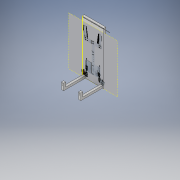
# Autodesk Inventor part: Pretend this is a harness
Saved by Autodesk Inventor 2018 (Build 220112000, 112)
## iProperties
Created: 2018-12-30
Part Number: Pretend this is a harness
Material: Generic
Document SubType Name: Modeling
Designer: maste
Density: 1 g/cm^3
Appearance: Default
Author: maste
Autodesk Inventor part; units mm, degrees
(part 1 of 4)
ref_plane "YZ Plane" through (0, 0, 0) normal (1, 0, 0) x (0, 1, 0)
ref_plane "XZ Plane" through (0, 0, 0) normal (0, 1, 0) x (-1, 0, 0)
ref_plane "XY Plane" through (0, 0, 0) normal (0, 0, 1) x (1, 0, 0)
sketch "Sketch1" plane through (0, 0, 0) normal (0, 0, 1) x (1, 0, 0)
  line L0 (0, 0) -> (250.7996, 0)
  line L1 (250.7996, 0) -> (250.7996, 609.6)
  line L2 (250.7996, 609.6) -> (0, 609.6)
  line L3 (0, 609.6) -> (0, 0)
  dimension "d0" = 250.7996
  dimension "d1" = 609.6
  constraints: 8 end point, 2 parallel, 1 horizontal, 1 perpendicular
  measures "d0" distance of L2.end L1.end
  measures "d1" distance of L1.end L0.end
extrude "Extrusion1" add sketch "Sketch1" along normal blind 25.4
sketch "Sketch2" plane through (0, 0, 25.4) normal (0, 0, 1) x (1, 0, 0)
  line L0 (0, 0) -> (25.4, 0) construction
  line L1 (0, 0) -> (250.7996, 0) construction
  line L2 (250.7996, 0) -> (225.3996, 0) construction
  line L3 (25.4, 0) -> (38.1, 0) construction
  line L4 (38.1, 0) -> (38.1, 25.4)
  line L5 (38.1, 25.4) -> (12.7, 25.4)
  line L6 (12.7, 25.4) -> (12.7, 0)
  line L7 (38.1, 0) -> (12.7, 0)
  line L8 (125.3998, 0) -> (125.3998, 65.8359) construction
  line L9 (250.7996, 0) -> (225.3996, 0) construction
  line L10 (250.7996, 0) -> (0, 0) construction
  line L11 (225.3996, 0) -> (212.6996, 0) construction
  line L12 (212.6996, 0) -> (212.6996, 25.4)
  line L13 (212.6996, 25.4) -> (238.0996, 25.4)
  line L14 (238.0996, 25.4) -> (238.0996, 0)
  line L15 (212.6996, 0) -> (238.0996, 0)
  dimension "d4" = 25.4
  dimension "d5" = 25.4
  dimension "d6" = 12.7
  dimension "d7" = 25.4
  dimension "d8" = 25.4
  constraints: 30 end point, 7 point on line, 6 symmetric about line, 3 perpendicular, 1 collinear, 1 midpoint, 1 vertical
  measures "d4" distance of L0.start L0.end
  measures "d5" distance of L1.end L2.end
  measures "d6" distance of L0.end L3.end
  measures "d7" distance of L3.end L4.end
  measures "d8" distance of L4.end L5.end
extrude "Extrusion2" add sketch "Sketch2" along normal blind 254
sketch "Sketch3" plane through (212.6996, 25.4, 25.4) normal (0, 1, 0) x (1, 0, 0)
  line L0 (-199.9996, -254) -> (-174.5996, -254) projected
  line L1 (-199.9996, -254) -> (-174.5996, -254)
  line L2 (-174.5996, -254) -> (-174.5996, -228.6)
  line L3 (-174.5996, -228.6) -> (-199.9996, -228.6)
  line L4 (-199.9996, -228.6) -> (-199.9996, -254)
  line L5 (0, -254) -> (25.4, -254) projected
  line L6 (25.4, 0) -> (25.4, -254) projected
  line L7 (0, -254) -> (25.4, -254)
  line L8 (25.4, -254) -> (25.4, -228.6)
  line L9 (25.4, -228.6) -> (0, -228.6)
  line L10 (0, -228.6) -> (0, -254)
  point P0 (-212.6996, 25.4)
  dimension "d11" = 25.4
  dimension "d12" = 25.4
  constraints: 16 end point, 4 parallel, 2 horizontal, 2 perpendicular, 2 point on line
  measures "d11" distance of L3.end L2.end
  measures "d12" distance of L2.end L1.end
extrude "Extrusion3" add sketch "Sketch3" along normal blind 50.8
sketch "Sketch4" plane through (0, 0, 279.4) normal (0, 0, 1) x (1, 0, 0)
  line L0 (38.1, 76.2) -> (12.7, 76.2) construction
  line L1 (25.4, 76.2) -> (25.4, 63.5) construction
  line L2 (25.4, 63.5) -> (25.4, 50.8) construction
  line L3 (38.1, 0) -> (212.6996, 0) construction
  line L4 (125.3998, 0) -> (125.3998, 112.4293) construction
  circle A0 centre (25.4, 50.8) radius 2.5797
  circle A1 centre (25.4, 63.5) radius 2.5797
  line L5 (212.6996, 76.2) -> (238.0996, 76.2) construction
  line L6 (225.3996, 76.2) -> (225.3996, 63.5) construction
  line L7 (225.3996, 63.5) -> (225.3996, 50.8) construction
  circle A2 centre (225.3996, 50.8) radius 2.5797
  circle A3 centre (225.3996, 63.5) radius 2.5797
  point P0 (0, 0)
  dimension "d15" = 12.7
  dimension "d16" = 12.7
  dimension "d17" = 5.1594
  constraints: 12 end point, 7 symmetric about line, 4 centre point, 4 coincident, 2 midpoint, 2 point on line, 2 vertical, 2 other
  measures "d15" distance of L1.start L1.end
  measures "d16" distance of L1.end L2.end
  measures "d17" diameter of A0
extrude "Extrusion4" cut sketch "Sketch4" against normal blind 50.8
sketch "Sketch5" plane through (0, 0, 25.4) normal (0, 0, 1) x (1, 0, 0)
  line L0 (0, 609.6) -> (0, 0) projected
  line L1 (-154.3078, 564.0513) -> (411.5707, 564.0513) construction
  line L2 (411.5707, 564.0513) -> (411.5707, -1.8272) construction
  line L3 (411.5707, -1.8272) -> (-154.3078, -1.8272) construction
  line L4 (-154.3078, -1.8272) -> (-154.3078, 564.0513) construction
  constraints: 2 end point, 2 other
sketch "Sketch6" plane through (0, 0, 25.4) normal (0, 0, 1) x (1, 0, 0)
  line L0 (9.9083, 603.5632) -> (254.2523, 603.5632) construction
  line L1 (254.2523, 603.5632) -> (254.2523, 561.4608) construction
  line L2 (254.2523, 561.4608) -> (9.9083, 561.4608) construction
  line L3 (9.9083, 561.4608) -> (9.9083, 603.5632) construction
  line L4 (11.9831, 600.3596) -> (11.5977, 600.3596)
  line L5 (11.5977, 600.3596) -> (11.5977, 601.6637)
  spline S0 degree 2 poles (11.5977, 601.6637) (11.5977, 601.8218) (11.5681, 602.0935) (11.5236, 602.175) knots 0 0 0 1 2 2 2
  spline S1 degree 2 poles (11.5236, 602.175) (11.4767, 602.2615) (11.3088, 602.3455) (11.1655, 602.3455) knots 0 0 0 1 2 2 2
  spline S2 degree 2 poles (11.1655, 602.3455) (11.0222, 602.3455) (10.7184, 602.1923) (10.5727, 602.0688) knots 0 0 0 1 2 2 2
  line L6 (10.5727, 602.0688) -> (10.5727, 600.3596)
  line L7 (10.5727, 600.3596) -> (10.1874, 600.3596)
  line L8 (10.1874, 600.3596) -> (10.1874, 603.5434)
  line L9 (10.1874, 603.5434) -> (10.5727, 603.5434)
  line L10 (10.5727, 603.5434) -> (10.5727, 602.3924)
  spline S3 degree 2 poles (10.5727, 602.3924) (10.7456, 602.548) (11.079, 602.711) (11.2668, 602.711) knots 0 0 0 1 2 2 2
  spline S4 degree 2 poles (11.2668, 602.711) (11.6027, 602.711) (11.9831, 602.2664) (11.9831, 601.844) knots 0 0 0 1 2 2 2
  line L11 (11.9831, 601.844) -> (11.9831, 600.3596)
  spline S5 degree 2 poles (13.2156, 600.3151) (12.9019, 600.3151) (12.5487, 600.6733) (12.5487, 601.061) knots 0 0 0 1 2 2 2
  line L12 (12.5487, 601.061) -> (12.5487, 602.3282)
  line L13 (12.5487, 602.3282) -> (12.2893, 602.3282)
  line L14 (12.2893, 602.3282) -> (12.2893, 602.6468)
  line L15 (12.2893, 602.6468) -> (12.5487, 602.6468)
  line L16 (12.5487, 602.6468) -> (12.5487, 603.3038)
  line L17 (12.5487, 603.3038) -> (12.934, 603.3038)
  line L18 (12.934, 603.3038) -> (12.934, 602.6468)
  line L19 (12.934, 602.6468) -> (13.6429, 602.6468)
  line L20 (13.6429, 602.6468) -> (13.6429, 602.3282)
  line L21 (13.6429, 602.3282) -> (12.934, 602.3282)
  line L22 (12.934, 602.3282) -> (12.934, 601.2389)
  spline S6 degree 2 poles (12.934, 601.2389) (12.934, 601.066) (12.9464, 600.8758) (12.9884, 600.7943) knots 0 0 0 1 2 2 2
  spline S7 degree 2 poles (12.9884, 600.7943) (13.0229, 600.7227) (13.1786, 600.651) (13.3119, 600.651) knots 0 0 0 1 2 2 2
  spline S8 degree 2 poles (13.3119, 600.651) (13.4058, 600.651) (13.5812, 600.7078) (13.6207, 600.7251) knots 0 0 0 1 2 2 2
  line L23 (13.6207, 600.7251) -> (13.6429, 600.7251)
  line L24 (13.6429, 600.7251) -> (13.6429, 600.3793)
  spline S9 degree 2 poles (13.6429, 600.3793) (13.5342, 600.3497) (13.3119, 600.3151) (13.2156, 600.3151) knots 0 0 0 1 2 2 2
  spline S10 degree 2 poles (14.6186, 600.3151) (14.3049, 600.3151) (13.9517, 600.6733) (13.9517, 601.061) knots 0 0 0 1 2 2 2
  line L25 (13.9517, 601.061) -> (13.9517, 602.3282)
  line L26 (13.9517, 602.3282) -> (13.6923, 602.3282)
  line L27 (13.6923, 602.3282) -> (13.6923, 602.6468)
  line L28 (13.6923, 602.6468) -> (13.9517, 602.6468)
  line L29 (13.9517, 602.6468) -> (13.9517, 603.3038)
  line L30 (13.9517, 603.3038) -> (14.337, 603.3038)
  line L31 (14.337, 603.3038) -> (14.337, 602.6468)
  line L32 (14.337, 602.6468) -> (15.0459, 602.6468)
  line L33 (15.0459, 602.6468) -> (15.0459, 602.3282)
  line L34 (15.0459, 602.3282) -> (14.337, 602.3282)
  line L35 (14.337, 602.3282) -> (14.337, 601.2389)
  spline S11 degree 2 poles (14.337, 601.2389) (14.337, 601.066) (14.3493, 600.8758) (14.3913, 600.7943) knots 0 0 0 1 2 2 2
  spline S12 degree 2 poles (14.3913, 600.7943) (14.4259, 600.7227) (14.5815, 600.651) (14.7149, 600.651) knots 0 0 0 1 2 2 2
  spline S13 degree 2 poles (14.7149, 600.651) (14.8088, 600.651) (14.9841, 600.7078) (15.0237, 600.7251) knots 0 0 0 1 2 2 2
  line L36 (15.0237, 600.7251) -> (15.0459, 600.7251)
  line L37 (15.0459, 600.7251) -> (15.0459, 600.3793)
  spline S14 degree 2 poles (15.0459, 600.3793) (14.9372, 600.3497) (14.7149, 600.3151) (14.6186, 600.3151) knots 0 0 0 1 2 2 2
  spline S15 degree 2 poles (17.2467, 601.5649) (17.2467, 600.9919) (16.7008, 600.3151) (16.2834, 600.3151) knots 0 0 0 1 2 2 2
  spline S16 degree 2 poles (16.2834, 600.3151) (16.1129, 600.3151) (15.8511, 600.3941) (15.7153, 600.4757) knots 0 0 0 1 2 2 2
  line L38 (15.7153, 600.4757) -> (15.7153, 599.5173)
  line L39 (15.7153, 599.5173) -> (15.3299, 599.5173)
  line L40 (15.3299, 599.5173) -> (15.3299, 602.6468)
  line L41 (15.3299, 602.6468) -> (15.7153, 602.6468)
  line L42 (15.7153, 602.6468) -> (15.7153, 602.4072)
  spline S17 degree 2 poles (15.7153, 602.4072) (15.8585, 602.5381) (16.2093, 602.711) (16.4143, 602.711) knots 0 0 0 1 2 2 2
  spline S18 degree 2 poles (16.4143, 602.711) (16.807, 602.711) (17.2467, 602.0886) (17.2467, 601.5649) knots 0 0 0 1 2 2 2
  spline S19 degree 2 poles (16.849, 601.5205) (16.849, 601.9132) (16.5995, 602.3455) (16.3204, 602.3455) knots 0 0 0 1 2 2 2
  spline S20 degree 2 poles (16.3204, 602.3455) (16.1574, 602.3455) (15.8511, 602.1997) (15.7153, 602.0861) knots 0 0 0 1 2 2 2
  line L43 (15.7153, 602.0861) -> (15.7153, 600.7869)
  spline S21 degree 2 poles (15.7153, 600.7869) (15.8659, 600.7152) (16.0808, 600.6609) (16.2191, 600.6609) knots 0 0 0 1 2 2 2
  spline S22 degree 2 poles (16.2191, 600.6609) (16.518, 600.6609) (16.849, 601.1006) (16.849, 601.5205) knots 0 0 0 1 2 2 2
  spline S23 degree 2 poles (18.2643, 600.3052) (18.0346, 600.3052) (17.6369, 600.4287) (17.506, 600.4979) knots 0 0 0 1 2 2 2
  line L44 (17.506, 600.4979) -> (17.506, 600.9301)
  line L45 (17.506, 600.9301) -> (17.5258, 600.9301)
  spline S24 degree 2 poles (17.5258, 600.9301) (17.5752, 600.8906) (17.7086, 600.7968) (17.8197, 600.7449) knots 0 0 0 1 2 2 2
  spline S25 degree 2 poles (17.8197, 600.7449) (17.916, 600.698) (18.1532, 600.6288) (18.2791, 600.6288) knots 0 0 0 1 2 2 2
  spline S26 degree 2 poles (18.2791, 600.6288) (18.3705, 600.6288) (18.5805, 600.6708) (18.6299, 600.7054) knots 0 0 0 1 2 2 2
  spline S27 degree 2 poles (18.6299, 600.7054) (18.7015, 600.7523) (18.7657, 600.8585) (18.7657, 600.9672) knots 0 0 0 1 2 2 2
  spline S28 degree 2 poles (18.7657, 600.9672) (18.7657, 601.103) (18.6175, 601.2438) (18.4273, 601.2908) knots 0 0 0 1 2 2 2
  spline S29 degree 2 poles (18.4273, 601.2908) (18.3532, 601.3081) (18.1161, 601.3575) (18.0148, 601.3846) knots 0 0 0 1 2 2 2
  spline S30 degree 2 poles (18.0148, 601.3846) (17.753, 601.4612) (17.5159, 601.7774) (17.5159, 602.0021) knots 0 0 0 1 2 2 2
  spline S31 degree 2 poles (17.5159, 602.0021) (17.5159, 602.3133) (17.9827, 602.7011) (18.3681, 602.7011) knots 0 0 0 1 2 2 2
  spline S32 degree 2 poles (18.3681, 602.7011) (18.5582, 602.7011) (18.9436, 602.6073) (19.0745, 602.5356) knots 0 0 0 1 2 2 2
  line L46 (19.0745, 602.5356) -> (19.0745, 602.1232)
  line L47 (19.0745, 602.1232) -> (19.0547, 602.1232)
  spline S33 degree 2 poles (19.0547, 602.1232) (18.9065, 602.2417) (18.5459, 602.3776) (18.3606, 602.3776) knots 0 0 0 1 2 2 2
  spline S34 degree 2 poles (18.3606, 602.3776) (18.1705, 602.3776) (17.9086, 602.217) (17.9086, 602.0565) knots 0 0 0 1 2 2 2
  spline S35 degree 2 poles (17.9086, 602.0565) (17.9086, 601.9107) (18.0642, 601.7699) (18.2371, 601.7255) knots 0 0 0 1 2 2 2
  spline S36 degree 2 poles (18.2371, 601.7255) (18.3211, 601.7033) (18.5335, 601.6588) (18.6496, 601.6316) knots 0 0 0 1 2 2 2
  spline S37 degree 2 poles (18.6496, 601.6316) (18.9016, 601.5674) (19.1585, 601.2735) (19.1585, 601.0191) knots 0 0 0 1 2 2 2
  spline S38 degree 2 poles (19.1585, 601.0191) (19.1585, 600.8709) (19.0424, 600.609) (18.9288, 600.5127) knots 0 0 0 1 2 2 2
  spline S39 degree 2 poles (18.9288, 600.5127) (18.8077, 600.4114) (18.499, 600.3052) (18.2643, 600.3052) knots 0 0 0 1 2 2 2
  line L48 (20.223, 600.3596) -> (19.734, 600.3596)
  line L49 (19.734, 600.3596) -> (19.734, 600.9425)
  line L50 (19.734, 600.9425) -> (20.223, 600.9425)
  line L51 (20.223, 600.9425) -> (20.223, 600.3596)
  line L52 (20.223, 602.0639) -> (19.734, 602.0639)
  line L53 (19.734, 602.0639) -> (19.734, 602.6468)
  line L54 (19.734, 602.6468) -> (20.223, 602.6468)
  line L55 (20.223, 602.6468) -> (20.223, 602.0639)
  line L56 (22.2089, 603.5434) -> (21.0159, 599.6976)
  line L57 (21.0159, 599.6976) -> (20.6701, 599.6976)
  line L58 (20.6701, 599.6976) -> (21.8582, 603.5434)
  line L59 (21.8582, 603.5434) -> (22.2089, 603.5434)
  line L60 (23.812, 603.5434) -> (22.619, 599.6976)
  line L61 (22.619, 599.6976) -> (22.2732, 599.6976)
  line L62 (22.2732, 599.6976) -> (23.4612, 603.5434)
  line L63 (23.4612, 603.5434) -> (23.812, 603.5434)
  line L64 (26.9761, 602.6468) -> (26.3956, 600.3596)
  line L65 (26.3956, 600.3596) -> (26.0399, 600.3596)
  line L66 (26.0399, 600.3596) -> (25.4817, 602.1232)
  line L67 (25.4817, 602.1232) -> (24.926, 600.3596)
  line L68 (24.926, 600.3596) -> (24.5727, 600.3596)
  line L69 (24.5727, 600.3596) -> (23.9873, 602.6468)
  line L70 (23.9873, 602.6468) -> (24.3875, 602.6468)
  line L71 (24.3875, 602.6468) -> (24.7926, 600.8758)
  line L72 (24.7926, 600.8758) -> (25.3335, 602.6468)
  line L73 (25.3335, 602.6468) -> (25.6521, 602.6468)
  line L74 (25.6521, 602.6468) -> (26.2079, 600.8758)
  line L75 (26.2079, 600.8758) -> (26.5883, 602.6468)
  line L76 (26.5883, 602.6468) -> (26.9761, 602.6468)
  line L77 (30.0858, 602.6468) -> (29.5054, 600.3596)
  line L78 (29.5054, 600.3596) -> (29.1497, 600.3596)
  line L79 (29.1497, 600.3596) -> (28.5915, 602.1232)
  line L80 (28.5915, 602.1232) -> (28.0357, 600.3596)
  line L81 (28.0357, 600.3596) -> (27.6825, 600.3596)
  line L82 (27.6825, 600.3596) -> (27.0971, 602.6468)
  line L83 (27.0971, 602.6468) -> (27.4972, 602.6468)
  line L84 (27.4972, 602.6468) -> (27.9023, 600.8758)
  line L85 (27.9023, 600.8758) -> (28.4433, 602.6468)
  line L86 (28.4433, 602.6468) -> (28.7619, 602.6468)
  line L87 (28.7619, 602.6468) -> (29.3176, 600.8758)
  line L88 (29.3176, 600.8758) -> (29.698, 602.6468)
  line L89 (29.698, 602.6468) -> (30.0858, 602.6468)
  line L90 (33.1956, 602.6468) -> (32.6151, 600.3596)
  line L91 (32.6151, 600.3596) -> (32.2594, 600.3596)
  line L92 (32.2594, 600.3596) -> (31.7012, 602.1232)
  line L93 (31.7012, 602.1232) -> (31.1455, 600.3596)
  line L94 (31.1455, 600.3596) -> (30.7922, 600.3596)
  line L95 (30.7922, 600.3596) -> (30.2068, 602.6468)
  line L96 (30.2068, 602.6468) -> (30.607, 602.6468)
  line L97 (30.607, 602.6468) -> (31.0121, 600.8758)
  line L98 (31.0121, 600.8758) -> (31.553, 602.6468)
  line L99 (31.553, 602.6468) -> (31.8716, 602.6468)
  line L100 (31.8716, 602.6468) -> (32.4274, 600.8758)
  line L101 (32.4274, 600.8758) -> (32.8078, 602.6468)
  line L102 (32.8078, 602.6468) -> (33.1956, 602.6468)
  line L103 (34.1317, 600.3596) -> (33.6426, 600.3596)
  line L104 (33.6426, 600.3596) -> (33.6426, 600.9425)
  line L105 (33.6426, 600.9425) -> (34.1317, 600.9425)
  line L106 (34.1317, 600.9425) -> (34.1317, 600.3596)
  spline S40 degree 2 poles (36.0781, 600.6016) (36.0311, 600.567) (35.8731, 600.4435) (35.799, 600.4065) knots 0 0 0 1 2 2 2
  spline S41 degree 2 poles (35.799, 600.4065) (35.6977, 600.3522) (35.5075, 600.2953) (35.3346, 600.2953) knots 0 0 0 1 2 2 2
  spline S42 degree 2 poles (35.3346, 600.2953) (35.1938, 600.2953) (34.9394, 600.4016) (34.8431, 600.4979) knots 0 0 0 1 2 2 2
  spline S43 degree 2 poles (34.8431, 600.4979) (34.7517, 600.5917) (34.6405, 600.8684) (34.6405, 601.0215) knots 0 0 0 1 2 2 2
  spline S44 degree 2 poles (34.6405, 601.0215) (34.6405, 601.2587) (34.8406, 601.5946) (35.058, 601.6909) knots 0 0 0 1 2 2 2
  spline S45 degree 2 poles (35.058, 601.6909) (35.2506, 601.7798) (35.7743, 601.8465) (36.0781, 601.8638) knots 0 0 0 1 2 2 2
  line L107 (36.0781, 601.8638) -> (36.0781, 601.9379)
  spline S46 degree 2 poles (36.0781, 601.9379) (36.0781, 602.0713) (35.9966, 602.2368) (35.9225, 602.2837) knots 0 0 0 1 2 2 2
  spline S47 degree 2 poles (35.9225, 602.2837) (35.8484, 602.3306) (35.6359, 602.3603) (35.5223, 602.3603) knots 0 0 0 1 2 2 2
  spline S48 degree 2 poles (35.5223, 602.3603) (35.3889, 602.3603) (35.0283, 602.2812) (34.848, 602.2047) knots 0 0 0 1 2 2 2
  line L108 (34.848, 602.2047) -> (34.8258, 602.2047)
  line L109 (34.8258, 602.2047) -> (34.8258, 602.5974)
  spline S49 degree 2 poles (34.8258, 602.5974) (34.932, 602.627) (35.3297, 602.7011) (35.5248, 602.7011) knots 0 0 0 1 2 2 2
  spline S50 degree 2 poles (35.5248, 602.7011) (35.7619, 602.7011) (36.0855, 602.627) (36.2139, 602.5307) knots 0 0 0 1 2 2 2
  spline S51 degree 2 poles (36.2139, 602.5307) (36.3399, 602.4368) (36.4634, 602.138) (36.4634, 601.9231) knots 0 0 0 1 2 2 2
  line L110 (36.4634, 601.9231) -> (36.4634, 600.3596)
  line L111 (36.4634, 600.3596) -> (36.0781, 600.3596)
  line L112 (36.0781, 600.3596) -> (36.0781, 600.6016)
  line L113 (36.0781, 600.9227) -> (36.0781, 601.5575)
  spline S52 degree 2 poles (36.0781, 601.5575) (35.9398, 601.5452) (35.5223, 601.5032) (35.3914, 601.4637) knots 0 0 0 1 2 2 2
  spline S53 degree 2 poles (35.3914, 601.4637) (35.2383, 601.4167) (35.0382, 601.2216) (35.0382, 601.0487) knots 0 0 0 1 2 2 2
  spline S54 degree 2 poles (35.0382, 601.0487) (35.0382, 600.8511) (35.2605, 600.651) (35.4729, 600.651) knots 0 0 0 1 2 2 2
  spline S55 degree 2 poles (35.4729, 600.651) (35.6532, 600.651) (35.9496, 600.8066) (36.0781, 600.9227) knots 0 0 0 1 2 2 2
  line L114 (39.5978, 600.3596) -> (39.5978, 601.6835)
  spline S56 degree 2 poles (39.5978, 601.6835) (39.5978, 601.8416) (39.5731, 602.1108) (39.5336, 602.1849) knots 0 0 0 1 2 2 2
  spline S57 degree 2 poles (39.5336, 602.1849) (39.4941, 602.2664) (39.3434, 602.3455) (39.2125, 602.3455) knots 0 0 0 1 2 2 2
  spline S58 degree 2 poles (39.2125, 602.3455) (39.094, 602.3455) (38.8223, 602.1997) (38.679, 602.0614) knots 0 0 0 1 2 2 2
  spline S59 degree 2 poles (38.679, 602.0614) (38.6815, 602.0268) (38.6864, 601.9305) (38.6864, 601.8663) knots 0 0 0 1 2 2 2
  line L115 (38.6864, 601.8663) -> (38.6864, 600.3596)
  line L116 (38.6864, 600.3596) -> (38.3011, 600.3596)
  line L117 (38.3011, 600.3596) -> (38.3011, 601.6835)
  spline S60 degree 2 poles (38.3011, 601.6835) (38.3011, 601.8416) (38.2764, 602.1108) (38.2369, 602.1849) knots 0 0 0 1 2 2 2
  spline S61 degree 2 poles (38.2369, 602.1849) (38.1973, 602.2664) (38.0467, 602.3455) (37.9158, 602.3455) knots 0 0 0 1 2 2 2
  spline S62 degree 2 poles (37.9158, 602.3455) (37.7923, 602.3455) (37.5181, 602.1898) (37.3897, 602.0688) knots 0 0 0 1 2 2 2
  line L118 (37.3897, 602.0688) -> (37.3897, 600.3596)
  line L119 (37.3897, 600.3596) -> (37.0043, 600.3596)
  line L120 (37.0043, 600.3596) -> (37.0043, 602.6468)
  line L121 (37.0043, 602.6468) -> (37.3897, 602.6468)
  line L122 (37.3897, 602.6468) -> (37.3897, 602.3949)
  spline S63 degree 2 poles (37.3897, 602.3949) (37.5403, 602.5455) (37.8367, 602.711) (38.0146, 602.711) knots 0 0 0 1 2 2 2
  spline S64 degree 2 poles (38.0146, 602.711) (38.2171, 602.711) (38.5308, 602.5258) (38.6123, 602.3158) knots 0 0 0 1 2 2 2
  spline S65 degree 2 poles (38.6123, 602.3158) (38.7877, 602.5109) (39.1187, 602.711) (39.3113, 602.711) knots 0 0 0 1 2 2 2
  spline S66 degree 2 poles (39.3113, 602.711) (39.4595, 602.711) (39.7016, 602.6196) (39.7905, 602.5159) knots 0 0 0 1 2 2 2
  spline S67 degree 2 poles (39.7905, 602.5159) (39.8819, 602.4121) (39.9832, 602.1009) (39.9832, 601.8663) knots 0 0 0 1 2 2 2
  line L123 (39.9832, 601.8663) -> (39.9832, 600.3596)
  line L124 (39.9832, 600.3596) -> (39.5978, 600.3596)
  spline S68 degree 2 poles (41.7986, 600.6016) (41.7517, 600.567) (41.5936, 600.4435) (41.5195, 600.4065) knots 0 0 0 1 2 2 2
  spline S69 degree 2 poles (41.5195, 600.4065) (41.4182, 600.3522) (41.2281, 600.2953) (41.0552, 600.2953) knots 0 0 0 1 2 2 2
  spline S70 degree 2 poles (41.0552, 600.2953) (40.9144, 600.2953) (40.66, 600.4016) (40.5636, 600.4979) knots 0 0 0 1 2 2 2
  spline S71 degree 2 poles (40.5636, 600.4979) (40.4722, 600.5917) (40.3611, 600.8684) (40.3611, 601.0215) knots 0 0 0 1 2 2 2
  spline S72 degree 2 poles (40.3611, 601.0215) (40.3611, 601.2587) (40.5612, 601.5946) (40.7785, 601.6909) knots 0 0 0 1 2 2 2
  spline S73 degree 2 poles (40.7785, 601.6909) (40.9712, 601.7798) (41.4948, 601.8465) (41.7986, 601.8638) knots 0 0 0 1 2 2 2
  line L125 (41.7986, 601.8638) -> (41.7986, 601.9379)
  spline S74 degree 2 poles (41.7986, 601.9379) (41.7986, 602.0713) (41.7171, 602.2368) (41.643, 602.2837) knots 0 0 0 1 2 2 2
  spline S75 degree 2 poles (41.643, 602.2837) (41.5689, 602.3306) (41.3565, 602.3603) (41.2429, 602.3603) knots 0 0 0 1 2 2 2
  spline S76 degree 2 poles (41.2429, 602.3603) (41.1095, 602.3603) (40.7489, 602.2812) (40.5686, 602.2047) knots 0 0 0 1 2 2 2
  line L126 (40.5686, 602.2047) -> (40.5463, 602.2047)
  line L127 (40.5463, 602.2047) -> (40.5463, 602.5974)
  spline S77 degree 2 poles (40.5463, 602.5974) (40.6525, 602.627) (41.0502, 602.7011) (41.2453, 602.7011) knots 0 0 0 1 2 2 2
  spline S78 degree 2 poles (41.2453, 602.7011) (41.4825, 602.7011) (41.806, 602.627) (41.9345, 602.5307) knots 0 0 0 1 2 2 2
  spline S79 degree 2 poles (41.9345, 602.5307) (42.0605, 602.4368) (42.184, 602.138) (42.184, 601.9231) knots 0 0 0 1 2 2 2
  line L128 (42.184, 601.9231) -> (42.184, 600.3596)
  line L129 (42.184, 600.3596) -> (41.7986, 600.3596)
  line L130 (41.7986, 600.3596) -> (41.7986, 600.6016)
  line L131 (41.7986, 600.9227) -> (41.7986, 601.5575)
  spline S80 degree 2 poles (41.7986, 601.5575) (41.6603, 601.5452) (41.2429, 601.5032) (41.112, 601.4637) knots 0 0 0 1 2 2 2
  spline S81 degree 2 poles (41.112, 601.4637) (40.9588, 601.4167) (40.7588, 601.2216) (40.7588, 601.0487) knots 0 0 0 1 2 2 2
  spline S82 degree 2 poles (40.7588, 601.0487) (40.7588, 600.8511) (40.9811, 600.651) (41.1935, 600.651) knots 0 0 0 1 2 2 2
  spline S83 degree 2 poles (41.1935, 600.651) (41.3738, 600.651) (41.6702, 600.8066) (41.7986, 600.9227) knots 0 0 0 1 2 2 2
  line L132 (44.2267, 600.3596) -> (42.547, 600.3596)
  line L133 (42.547, 600.3596) -> (42.547, 600.6461)
  line L134 (42.547, 600.6461) -> (43.7425, 602.3306)
  line L135 (43.7425, 602.3306) -> (42.5964, 602.3306)
  line L136 (42.5964, 602.3306) -> (42.5964, 602.6468)
  line L137 (42.5964, 602.6468) -> (44.2044, 602.6468)
  line L138 (44.2044, 602.6468) -> (44.2044, 602.3726)
  line L139 (44.2044, 602.3726) -> (43.004, 600.6831)
  line L140 (43.004, 600.6831) -> (44.2267, 600.6831)
  line L141 (44.2267, 600.6831) -> (44.2267, 600.3596)
  spline S84 degree 2 poles (46.467, 601.5032) (46.467, 600.9252) (45.9112, 600.2953) (45.4468, 600.2953) knots 0 0 0 1 2 2 2
  spline S85 degree 2 poles (45.4468, 600.2953) (44.9701, 600.2953) (44.4243, 600.945) (44.4243, 601.5032) knots 0 0 0 1 2 2 2
  spline S86 degree 2 poles (44.4243, 601.5032) (44.4243, 602.0762) (44.9874, 602.711) (45.4468, 602.711) knots 0 0 0 1 2 2 2
  spline S87 degree 2 poles (45.4468, 602.711) (45.9112, 602.711) (46.467, 602.0787) (46.467, 601.5032) knots 0 0 0 1 2 2 2
  spline S88 degree 2 poles (46.0693, 601.5032) (46.0693, 601.9478) (45.7457, 602.38) (45.4468, 602.38) knots 0 0 0 1 2 2 2
  spline S89 degree 2 poles (45.4468, 602.38) (45.148, 602.38) (44.8219, 601.9478) (44.8219, 601.5032) knots 0 0 0 1 2 2 2
  spline S90 degree 2 poles (44.8219, 601.5032) (44.8219, 601.0709) (45.148, 600.6263) (45.4468, 600.6263) knots 0 0 0 1 2 2 2
  spline S91 degree 2 poles (45.4468, 600.6263) (45.7432, 600.6263) (46.0693, 601.0635) (46.0693, 601.5032) knots 0 0 0 1 2 2 2
  line L142 (48.6579, 600.3596) -> (48.2725, 600.3596)
  line L143 (48.2725, 600.3596) -> (48.2725, 601.6637)
  spline S92 degree 2 poles (48.2725, 601.6637) (48.2725, 601.8218) (48.2429, 602.0935) (48.1984, 602.175) knots 0 0 0 1 2 2 2
  spline S93 degree 2 poles (48.1984, 602.175) (48.1515, 602.2615) (47.9836, 602.3455) (47.8403, 602.3455) knots 0 0 0 1 2 2 2
  spline S94 degree 2 poles (47.8403, 602.3455) (47.697, 602.3455) (47.3932, 602.1923) (47.2475, 602.0688) knots 0 0 0 1 2 2 2
  line L144 (47.2475, 602.0688) -> (47.2475, 600.3596)
  line L145 (47.2475, 600.3596) -> (46.8622, 600.3596)
  line L146 (46.8622, 600.3596) -> (46.8622, 602.6468)
  line L147 (46.8622, 602.6468) -> (47.2475, 602.6468)
  line L148 (47.2475, 602.6468) -> (47.2475, 602.3924)
  spline S95 degree 2 poles (47.2475, 602.3924) (47.4204, 602.548) (47.7538, 602.711) (47.9416, 602.711) knots 0 0 0 1 2 2 2
  spline S96 degree 2 poles (47.9416, 602.711) (48.2775, 602.711) (48.6579, 602.2664) (48.6579, 601.844) knots 0 0 0 1 2 2 2
  line L149 (48.6579, 601.844) -> (48.6579, 600.3596)
  line L150 (49.7965, 600.3596) -> (49.3075, 600.3596)
  line L151 (49.3075, 600.3596) -> (49.3075, 600.9425)
  line L152 (49.3075, 600.9425) -> (49.7965, 600.9425)
  line L153 (49.7965, 600.9425) -> (49.7965, 600.3596)
  spline S97 degree 2 poles (51.3774, 600.3077) (51.1402, 600.3077) (50.7475, 600.4534) (50.6067, 600.6016) knots 0 0 0 1 2 2 2
  spline S98 degree 2 poles (50.6067, 600.6016) (50.4659, 600.7474) (50.3103, 601.1969) (50.3103, 601.4982) knots 0 0 0 1 2 2 2
  spline S99 degree 2 poles (50.3103, 601.4982) (50.3103, 601.7996) (50.4709, 602.2392) (50.6067, 602.3874) knots 0 0 0 1 2 2 2
  spline S100 degree 2 poles (50.6067, 602.3874) (50.7426, 602.5381) (51.1452, 602.6987) (51.3774, 602.6987) knots 0 0 0 1 2 2 2
  spline S101 degree 2 poles (51.3774, 602.6987) (51.5651, 602.6987) (51.9158, 602.5925) (52.0517, 602.5233) knots 0 0 0 1 2 2 2
  line L154 (52.0517, 602.5233) -> (52.0517, 602.091)
  line L155 (52.0517, 602.091) -> (52.0294, 602.091)
  spline S102 degree 2 poles (52.0294, 602.091) (51.9874, 602.1256) (51.859, 602.2145) (51.7676, 602.2615) knots 0 0 0 1 2 2 2
  spline S103 degree 2 poles (51.7676, 602.2615) (51.6861, 602.301) (51.4687, 602.3627) (51.3699, 602.3627) knots 0 0 0 1 2 2 2
  spline S104 degree 2 poles (51.3699, 602.3627) (51.0711, 602.3627) (50.708, 601.9107) (50.708, 601.4982) knots 0 0 0 1 2 2 2
  spline S105 degree 2 poles (50.708, 601.4982) (50.708, 601.0956) (51.0587, 600.6436) (51.3699, 600.6436) knots 0 0 0 1 2 2 2
  spline S106 degree 2 poles (51.3699, 600.6436) (51.5577, 600.6436) (51.8985, 600.7992) (52.0294, 600.9203) knots 0 0 0 1 2 2 2
  line L156 (52.0294, 600.9203) -> (52.0517, 600.9203)
  line L157 (52.0517, 600.9203) -> (52.0517, 600.488)
  spline S107 degree 2 poles (52.0517, 600.488) (51.9949, 600.4608) (51.822, 600.3843) (51.7528, 600.367) knots 0 0 0 1 2 2 2
  spline S108 degree 2 poles (51.7528, 600.367) (51.654, 600.3373) (51.4984, 600.3077) (51.3774, 600.3077) knots 0 0 0 1 2 2 2
  spline S109 degree 2 poles (54.2821, 601.5032) (54.2821, 600.9252) (53.7263, 600.2953) (53.262, 600.2953) knots 0 0 0 1 2 2 2
  spline S110 degree 2 poles (53.262, 600.2953) (52.7853, 600.2953) (52.2394, 600.945) (52.2394, 601.5032) knots 0 0 0 1 2 2 2
  spline S111 degree 2 poles (52.2394, 601.5032) (52.2394, 602.0762) (52.8026, 602.711) (53.262, 602.711) knots 0 0 0 1 2 2 2
  spline S112 degree 2 poles (53.262, 602.711) (53.7263, 602.711) (54.2821, 602.0787) (54.2821, 601.5032) knots 0 0 0 1 2 2 2
  spline S113 degree 2 poles (53.8844, 601.5032) (53.8844, 601.9478) (53.5608, 602.38) (53.262, 602.38) knots 0 0 0 1 2 2 2
  spline S114 degree 2 poles (53.262, 602.38) (52.9631, 602.38) (52.6371, 601.9478) (52.6371, 601.5032) knots 0 0 0 1 2 2 2
  spline S115 degree 2 poles (52.6371, 601.5032) (52.6371, 601.0709) (52.9631, 600.6263) (53.262, 600.6263) knots 0 0 0 1 2 2 2
  spline S116 degree 2 poles (53.262, 600.6263) (53.5584, 600.6263) (53.8844, 601.0635) (53.8844, 601.5032) knots 0 0 0 1 2 2 2
  line L158 (57.2708, 600.3596) -> (57.2708, 601.6835)
  spline S117 degree 2 poles (57.2708, 601.6835) (57.2708, 601.8416) (57.2461, 602.1108) (57.2066, 602.1849) knots 0 0 0 1 2 2 2
  spline S118 degree 2 poles (57.2066, 602.1849) (57.1671, 602.2664) (57.0164, 602.3455) (56.8855, 602.3455) knots 0 0 0 1 2 2 2
  spline S119 degree 2 poles (56.8855, 602.3455) (56.7669, 602.3455) (56.4952, 602.1997) (56.352, 602.0614) knots 0 0 0 1 2 2 2
  spline S120 degree 2 poles (56.352, 602.0614) (56.3544, 602.0268) (56.3594, 601.9305) (56.3594, 601.8663) knots 0 0 0 1 2 2 2
  line L159 (56.3594, 601.8663) -> (56.3594, 600.3596)
  line L160 (56.3594, 600.3596) -> (55.9741, 600.3596)
  line L161 (55.9741, 600.3596) -> (55.9741, 601.6835)
  spline S121 degree 2 poles (55.9741, 601.6835) (55.9741, 601.8416) (55.9494, 602.1108) (55.9098, 602.1849) knots 0 0 0 1 2 2 2
  spline S122 degree 2 poles (55.9098, 602.1849) (55.8703, 602.2664) (55.7196, 602.3455) (55.5887, 602.3455) knots 0 0 0 1 2 2 2
  spline S123 degree 2 poles (55.5887, 602.3455) (55.4652, 602.3455) (55.1911, 602.1898) (55.0626, 602.0688) knots 0 0 0 1 2 2 2
  line L162 (55.0626, 602.0688) -> (55.0626, 600.3596)
  line L163 (55.0626, 600.3596) -> (54.6773, 600.3596)
  line L164 (54.6773, 600.3596) -> (54.6773, 602.6468)
  line L165 (54.6773, 602.6468) -> (55.0626, 602.6468)
  line L166 (55.0626, 602.6468) -> (55.0626, 602.3949)
  spline S124 degree 2 poles (55.0626, 602.3949) (55.2133, 602.5455) (55.5097, 602.711) (55.6875, 602.711) knots 0 0 0 1 2 2 2
  spline S125 degree 2 poles (55.6875, 602.711) (55.8901, 602.711) (56.2038, 602.5258) (56.2853, 602.3158) knots 0 0 0 1 2 2 2
  spline S126 degree 2 poles (56.2853, 602.3158) (56.4606, 602.5109) (56.7916, 602.711) (56.9843, 602.711) knots 0 0 0 1 2 2 2
  spline S127 degree 2 poles (56.9843, 602.711) (57.1325, 602.711) (57.3746, 602.6196) (57.4635, 602.5159) knots 0 0 0 1 2 2 2
  spline S128 degree 2 poles (57.4635, 602.5159) (57.5549, 602.4121) (57.6561, 602.1009) (57.6561, 601.8663) knots 0 0 0 1 2 2 2
  line L167 (57.6561, 601.8663) -> (57.6561, 600.3596)
  line L168 (57.6561, 600.3596) -> (57.2708, 600.3596)
  line L169 (59.4074, 603.5434) -> (58.2144, 599.6976)
  line L170 (58.2144, 599.6976) -> (57.8686, 599.6976)
  line L171 (57.8686, 599.6976) -> (59.0566, 603.5434)
  line L172 (59.0566, 603.5434) -> (59.4074, 603.5434)
  line L173 (60.1928, 600.3596) -> (59.8075, 600.3596)
  line L174 (59.8075, 600.3596) -> (59.8075, 603.5434)
  line L175 (59.8075, 603.5434) -> (60.1928, 603.5434)
  line L176 (60.1928, 603.5434) -> (60.1928, 600.3596)
  spline S129 degree 2 poles (62.6382, 601.5032) (62.6382, 600.9252) (62.0824, 600.2953) (61.618, 600.2953) knots 0 0 0 1 2 2 2
  spline S130 degree 2 poles (61.618, 600.2953) (61.1413, 600.2953) (60.5955, 600.945) (60.5955, 601.5032) knots 0 0 0 1 2 2 2
  spline S131 degree 2 poles (60.5955, 601.5032) (60.5955, 602.0762) (61.1586, 602.711) (61.618, 602.711) knots 0 0 0 1 2 2 2
  spline S132 degree 2 poles (61.618, 602.711) (62.0824, 602.711) (62.6382, 602.0787) (62.6382, 601.5032) knots 0 0 0 1 2 2 2
  spline S133 degree 2 poles (62.2405, 601.5032) (62.2405, 601.9478) (61.9169, 602.38) (61.618, 602.38) knots 0 0 0 1 2 2 2
  spline S134 degree 2 poles (61.618, 602.38) (61.3192, 602.38) (60.9931, 601.9478) (60.9931, 601.5032) knots 0 0 0 1 2 2 2
  spline S135 degree 2 poles (60.9931, 601.5032) (60.9931, 601.0709) (61.3192, 600.6263) (61.618, 600.6263) knots 0 0 0 1 2 2 2
  spline S136 degree 2 poles (61.618, 600.6263) (61.9144, 600.6263) (62.2405, 601.0635) (62.2405, 601.5032) knots 0 0 0 1 2 2 2
  line L177 (64.8291, 602.6468) -> (63.967, 600.3596)
  line L178 (63.967, 600.3596) -> (63.6212, 600.3596)
  line L179 (63.6212, 600.3596) -> (62.7666, 602.6468)
  line L180 (62.7666, 602.6468) -> (63.184, 602.6468)
  line L181 (63.184, 602.6468) -> (63.8089, 600.8857)
  line L182 (63.8089, 600.8857) -> (64.4289, 602.6468)
  line L183 (64.4289, 602.6468) -> (64.8291, 602.6468)
  spline S137 degree 2 poles (66.1135, 600.3077) (65.5651, 600.3077) (64.9624, 600.9227) (64.9624, 601.4908) knots 0 0 0 1 2 2 2
  spline S138 degree 2 poles (64.9624, 601.4908) (64.9624, 602.0491) (65.5478, 602.711) (66.0196, 602.711) knots 0 0 0 1 2 2 2
  spline S139 degree 2 poles (66.0196, 602.711) (66.232, 602.711) (66.5605, 602.5875) (66.6816, 602.4566) knots 0 0 0 1 2 2 2
  spline S140 degree 2 poles (66.6816, 602.4566) (66.8051, 602.3257) (66.936, 601.9478) (66.936, 601.6736) knots 0 0 0 1 2 2 2
  line L184 (66.936, 601.6736) -> (66.936, 601.4637)
  line L185 (66.936, 601.4637) -> (65.3527, 601.4637)
  spline S141 degree 2 poles (65.3527, 601.4637) (65.3527, 601.066) (65.7528, 600.6436) (66.1085, 600.6436) knots 0 0 0 1 2 2 2
  spline S142 degree 2 poles (66.1085, 600.6436) (66.2345, 600.6436) (66.479, 600.7004) (66.5778, 600.7449) knots 0 0 0 1 2 2 2
  spline S143 degree 2 poles (66.5778, 600.7449) (66.6816, 600.7943) (66.8248, 600.8807) (66.8718, 600.9203) knots 0 0 0 1 2 2 2
  line L186 (66.8718, 600.9203) -> (66.894, 600.9203)
  line L187 (66.894, 600.9203) -> (66.894, 600.5004)
  spline S144 degree 2 poles (66.894, 600.5004) (66.8273, 600.4732) (66.6248, 600.3941) (66.5457, 600.3719) knots 0 0 0 1 2 2 2
  spline S145 degree 2 poles (66.5457, 600.3719) (66.4346, 600.3398) (66.2518, 600.3077) (66.1135, 600.3077) knots 0 0 0 1 2 2 2
  spline S146 degree 2 poles (66.5605, 601.7576) (66.5556, 601.9132) (66.4914, 602.1404) (66.4296, 602.217) knots 0 0 0 1 2 2 2
  spline S147 degree 2 poles (66.4296, 602.217) (66.3629, 602.3035) (66.153, 602.3949) (65.9974, 602.3949) knots 0 0 0 1 2 2 2
  spline S148 degree 2 poles (65.9974, 602.3949) (65.8442, 602.3949) (65.6293, 602.3035) (65.5404, 602.2145) knots 0 0 0 1 2 2 2
  spline S149 degree 2 poles (65.5404, 602.2145) (65.454, 602.1232) (65.3651, 601.9033) (65.3527, 601.7576) knots 0 0 0 1 2 2 2
  line L188 (65.3527, 601.7576) -> (66.5605, 601.7576)
  line L189 (68.539, 602.2343) -> (68.5193, 602.2343)
  spline S150 degree 2 poles (68.5193, 602.2343) (68.4748, 602.2467) (68.3785, 602.2516) (68.3118, 602.2516) knots 0 0 0 1 2 2 2
  spline S151 degree 2 poles (68.3118, 602.2516) (68.1562, 602.2516) (67.8499, 602.1157) (67.7116, 601.9824) knots 0 0 0 1 2 2 2
  line L190 (67.7116, 601.9824) -> (67.7116, 600.3596)
  line L191 (67.7116, 600.3596) -> (67.3262, 600.3596)
  line L192 (67.3262, 600.3596) -> (67.3262, 602.6468)
  line L193 (67.3262, 602.6468) -> (67.7116, 602.6468)
  line L194 (67.7116, 602.6468) -> (67.7116, 602.3059)
  spline S152 degree 2 poles (67.7116, 602.3059) (67.9215, 602.4937) (68.2352, 602.6468) (68.3834, 602.6468) knots 0 0 0 1 2 2 2
  spline S153 degree 2 poles (68.3834, 602.6468) (68.4427, 602.6468) (68.502, 602.6419) (68.539, 602.6344) knots 0 0 0 1 2 2 2
  line L195 (68.539, 602.6344) -> (68.539, 602.2343)
  line L196 (71.4314, 600.3596) -> (71.4314, 601.6835)
  spline S154 degree 2 poles (71.4314, 601.6835) (71.4314, 601.8416) (71.4067, 602.1108) (71.3672, 602.1849) knots 0 0 0 1 2 2 2
  spline S155 degree 2 poles (71.3672, 602.1849) (71.3277, 602.2664) (71.177, 602.3455) (71.0461, 602.3455) knots 0 0 0 1 2 2 2
  spline S156 degree 2 poles (71.0461, 602.3455) (70.9275, 602.3455) (70.6558, 602.1997) (70.5126, 602.0614) knots 0 0 0 1 2 2 2
  spline S157 degree 2 poles (70.5126, 602.0614) (70.515, 602.0268) (70.52, 601.9305) (70.52, 601.8663) knots 0 0 0 1 2 2 2
  line L197 (70.52, 601.8663) -> (70.52, 600.3596)
  line L198 (70.52, 600.3596) -> (70.1347, 600.3596)
  line L199 (70.1347, 600.3596) -> (70.1347, 601.6835)
  spline S158 degree 2 poles (70.1347, 601.6835) (70.1347, 601.8416) (70.11, 602.1108) (70.0704, 602.1849) knots 0 0 0 1 2 2 2
  spline S159 degree 2 poles (70.0704, 602.1849) (70.0309, 602.2664) (69.8802, 602.3455) (69.7493, 602.3455) knots 0 0 0 1 2 2 2
  spline S160 degree 2 poles (69.7493, 602.3455) (69.6258, 602.3455) (69.3517, 602.1898) (69.2232, 602.0688) knots 0 0 0 1 2 2 2
  line L200 (69.2232, 602.0688) -> (69.2232, 600.3596)
  line L201 (69.2232, 600.3596) -> (68.8379, 600.3596)
  line L202 (68.8379, 600.3596) -> (68.8379, 602.6468)
  line L203 (68.8379, 602.6468) -> (69.2232, 602.6468)
  line L204 (69.2232, 602.6468) -> (69.2232, 602.3949)
  spline S161 degree 2 poles (69.2232, 602.3949) (69.3739, 602.5455) (69.6703, 602.711) (69.8481, 602.711) knots 0 0 0 1 2 2 2
  spline S162 degree 2 poles (69.8481, 602.711) (70.0507, 602.711) (70.3644, 602.5258) (70.4459, 602.3158) knots 0 0 0 1 2 2 2
  spline S163 degree 2 poles (70.4459, 602.3158) (70.6213, 602.5109) (70.9522, 602.711) (71.1449, 602.711) knots 0 0 0 1 2 2 2
  spline S164 degree 2 poles (71.1449, 602.711) (71.2931, 602.711) (71.5352, 602.6196) (71.6241, 602.5159) knots 0 0 0 1 2 2 2
  spline S165 degree 2 poles (71.6241, 602.5159) (71.7155, 602.4121) (71.8167, 602.1009) (71.8167, 601.8663) knots 0 0 0 1 2 2 2
  line L205 (71.8167, 601.8663) -> (71.8167, 600.3596)
  line L206 (71.8167, 600.3596) -> (71.4314, 600.3596)
  line L207 (74.1361, 600.3596) -> (73.7508, 600.3596)
  line L208 (73.7508, 600.3596) -> (73.7508, 600.6115)
  spline S166 degree 2 poles (73.7508, 600.6115) (73.5729, 600.4559) (73.2543, 600.2953) (73.0567, 600.2953) knots 0 0 0 1 2 2 2
  spline S167 degree 2 poles (73.0567, 600.2953) (72.9085, 600.2953) (72.6442, 600.3941) (72.5479, 600.5004) knots 0 0 0 1 2 2 2
  spline S168 degree 2 poles (72.5479, 600.5004) (72.4491, 600.6066) (72.3404, 600.9301) (72.3404, 601.1623) knots 0 0 0 1 2 2 2
  line L209 (72.3404, 601.1623) -> (72.3404, 602.6468)
  line L210 (72.3404, 602.6468) -> (72.7257, 602.6468)
  line L211 (72.7257, 602.6468) -> (72.7257, 601.3426)
  spline S169 degree 2 poles (72.7257, 601.3426) (72.7257, 601.1598) (72.7529, 600.9203) (72.7998, 600.8313) knots 0 0 0 1 2 2 2
  spline S170 degree 2 poles (72.7998, 600.8313) (72.8467, 600.7424) (73.0073, 600.6609) (73.158, 600.6609) knots 0 0 0 1 2 2 2
  spline S171 degree 2 poles (73.158, 600.6609) (73.2987, 600.6609) (73.6174, 600.8215) (73.7508, 600.9375) knots 0 0 0 1 2 2 2
  line L212 (73.7508, 600.9375) -> (73.7508, 602.6468)
  line L213 (73.7508, 602.6468) -> (74.1361, 602.6468)
  line L214 (74.1361, 602.6468) -> (74.1361, 600.3596)
  spline S172 degree 2 poles (75.3118, 600.3052) (75.0821, 600.3052) (74.6844, 600.4287) (74.5535, 600.4979) knots 0 0 0 1 2 2 2
  line L215 (74.5535, 600.4979) -> (74.5535, 600.9301)
  line L216 (74.5535, 600.9301) -> (74.5733, 600.9301)
  spline S173 degree 2 poles (74.5733, 600.9301) (74.6227, 600.8906) (74.7561, 600.7968) (74.8672, 600.7449) knots 0 0 0 1 2 2 2
  spline S174 degree 2 poles (74.8672, 600.7449) (74.9635, 600.698) (75.2007, 600.6288) (75.3266, 600.6288) knots 0 0 0 1 2 2 2
  spline S175 degree 2 poles (75.3266, 600.6288) (75.418, 600.6288) (75.628, 600.6708) (75.6774, 600.7054) knots 0 0 0 1 2 2 2
  spline S176 degree 2 poles (75.6774, 600.7054) (75.749, 600.7523) (75.8132, 600.8585) (75.8132, 600.9672) knots 0 0 0 1 2 2 2
  spline S177 degree 2 poles (75.8132, 600.9672) (75.8132, 601.103) (75.665, 601.2438) (75.4748, 601.2908) knots 0 0 0 1 2 2 2
  spline S178 degree 2 poles (75.4748, 601.2908) (75.4007, 601.3081) (75.1636, 601.3575) (75.0623, 601.3846) knots 0 0 0 1 2 2 2
  spline S179 degree 2 poles (75.0623, 601.3846) (74.8005, 601.4612) (74.5634, 601.7774) (74.5634, 602.0021) knots 0 0 0 1 2 2 2
  spline S180 degree 2 poles (74.5634, 602.0021) (74.5634, 602.3133) (75.0302, 602.7011) (75.4156, 602.7011) knots 0 0 0 1 2 2 2
  spline S181 degree 2 poles (75.4156, 602.7011) (75.6057, 602.7011) (75.9911, 602.6073) (76.122, 602.5356) knots 0 0 0 1 2 2 2
  line L217 (76.122, 602.5356) -> (76.122, 602.1232)
  line L218 (76.122, 602.1232) -> (76.1022, 602.1232)
  spline S182 degree 2 poles (76.1022, 602.1232) (75.954, 602.2417) (75.5934, 602.3776) (75.4081, 602.3776) knots 0 0 0 1 2 2 2
  spline S183 degree 2 poles (75.4081, 602.3776) (75.218, 602.3776) (74.9561, 602.217) (74.9561, 602.0565) knots 0 0 0 1 2 2 2
  spline S184 degree 2 poles (74.9561, 602.0565) (74.9561, 601.9107) (75.1117, 601.7699) (75.2846, 601.7255) knots 0 0 0 1 2 2 2
  spline S185 degree 2 poles (75.2846, 601.7255) (75.3686, 601.7033) (75.581, 601.6588) (75.6971, 601.6316) knots 0 0 0 1 2 2 2
  spline S186 degree 2 poles (75.6971, 601.6316) (75.9491, 601.5674) (76.206, 601.2735) (76.206, 601.0191) knots 0 0 0 1 2 2 2
  spline S187 degree 2 poles (76.206, 601.0191) (76.206, 600.8709) (76.0899, 600.609) (75.9762, 600.5127) knots 0 0 0 1 2 2 2
  spline S188 degree 2 poles (75.9762, 600.5127) (75.8552, 600.4114) (75.5465, 600.3052) (75.3118, 600.3052) knots 0 0 0 1 2 2 2
  line L219 (76.9568, 600.3596) -> (76.5715, 600.3596)
  line L220 (76.5715, 600.3596) -> (76.5715, 602.6468)
  line L221 (76.5715, 602.6468) -> (76.9568, 602.6468)
  line L222 (76.9568, 602.6468) -> (76.9568, 600.3596)
  line L223 (76.984, 603.0272) -> (76.5468, 603.0272)
  line L224 (76.5468, 603.0272) -> (76.5468, 603.4273)
  line L225 (76.5468, 603.4273) -> (76.984, 603.4273)
  line L226 (76.984, 603.4273) -> (76.984, 603.0272)
  spline S189 degree 2 poles (78.4314, 600.3077) (78.1943, 600.3077) (77.8016, 600.4534) (77.6608, 600.6016) knots 0 0 0 1 2 2 2
  spline S190 degree 2 poles (77.6608, 600.6016) (77.52, 600.7474) (77.3644, 601.1969) (77.3644, 601.4982) knots 0 0 0 1 2 2 2
  spline S191 degree 2 poles (77.3644, 601.4982) (77.3644, 601.7996) (77.5249, 602.2392) (77.6608, 602.3874) knots 0 0 0 1 2 2 2
  spline S192 degree 2 poles (77.6608, 602.3874) (77.7966, 602.5381) (78.1993, 602.6987) (78.4314, 602.6987) knots 0 0 0 1 2 2 2
  spline S193 degree 2 poles (78.4314, 602.6987) (78.6192, 602.6987) (78.9699, 602.5925) (79.1058, 602.5233) knots 0 0 0 1 2 2 2
  line L227 (79.1058, 602.5233) -> (79.1058, 602.091)
  line L228 (79.1058, 602.091) -> (79.0835, 602.091)
  spline S194 degree 2 poles (79.0835, 602.091) (79.0415, 602.1256) (78.9131, 602.2145) (78.8217, 602.2615) knots 0 0 0 1 2 2 2
  spline S195 degree 2 poles (78.8217, 602.2615) (78.7402, 602.301) (78.5228, 602.3627) (78.424, 602.3627) knots 0 0 0 1 2 2 2
  spline S196 degree 2 poles (78.424, 602.3627) (78.1252, 602.3627) (77.7621, 601.9107) (77.7621, 601.4982) knots 0 0 0 1 2 2 2
  spline S197 degree 2 poles (77.7621, 601.4982) (77.7621, 601.0956) (78.1128, 600.6436) (78.424, 600.6436) knots 0 0 0 1 2 2 2
  spline S198 degree 2 poles (78.424, 600.6436) (78.6118, 600.6436) (78.9526, 600.7992) (79.0835, 600.9203) knots 0 0 0 1 2 2 2
  line L229 (79.0835, 600.9203) -> (79.1058, 600.9203)
  line L230 (79.1058, 600.9203) -> (79.1058, 600.488)
  spline S199 degree 2 poles (79.1058, 600.488) (79.0489, 600.4608) (78.876, 600.3843) (78.8069, 600.367) knots 0 0 0 1 2 2 2
  spline S200 degree 2 poles (78.8069, 600.367) (78.7081, 600.3373) (78.5525, 600.3077) (78.4314, 600.3077) knots 0 0 0 1 2 2 2
  line L231 (80.5161, 601.5081) -> (79.3626, 601.5081)
  line L232 (79.3626, 601.5081) -> (79.3626, 601.8786)
  line L233 (79.3626, 601.8786) -> (80.5161, 601.8786)
  line L234 (80.5161, 601.8786) -> (80.5161, 601.5081)
  spline S201 degree 2 poles (82.9343, 602.4887) (82.9343, 602.2911) (82.7935, 601.9354) (82.6675, 601.8119) knots 0 0 0 1 2 2 2
  spline S202 degree 2 poles (82.6675, 601.8119) (82.5094, 601.6563) (82.0821, 601.4958) (81.7561, 601.4958) knots 0 0 0 1 2 2 2
  line L235 (81.7561, 601.4958) -> (81.4128, 601.4958)
  line L236 (81.4128, 601.4958) -> (81.4128, 600.3596)
  line L237 (81.4128, 600.3596) -> (81.0077, 600.3596)
  line L238 (81.0077, 600.3596) -> (81.0077, 603.4076)
  line L239 (81.0077, 603.4076) -> (81.7734, 603.4076)
  spline S203 degree 2 poles (81.7734, 603.4076) (82.0451, 603.4076) (82.4255, 603.3186) (82.5712, 603.2174) knots 0 0 0 1 2 2 2
  spline S204 degree 2 poles (82.5712, 603.2174) (82.7416, 603.1013) (82.9343, 602.7431) (82.9343, 602.4887) knots 0 0 0 1 2 2 2
  spline S205 degree 2 poles (82.5119, 602.4764) (82.5119, 602.6344) (82.4032, 602.8666) (82.2921, 602.9407) knots 0 0 0 1 2 2 2
  spline S206 degree 2 poles (82.2921, 602.9407) (82.1957, 603.005) (81.9389, 603.0568) (81.7487, 603.0568) knots 0 0 0 1 2 2 2
  line L240 (81.7487, 603.0568) -> (81.4128, 603.0568)
  line L241 (81.4128, 603.0568) -> (81.4128, 601.8416)
  line L242 (81.4128, 601.8416) -> (81.6894, 601.8416)
  spline S207 degree 2 poles (81.6894, 601.8416) (81.9364, 601.8416) (82.2402, 601.9206) (82.339, 602.0244) knots 0 0 0 1 2 2 2
  spline S208 degree 2 poles (82.339, 602.0244) (82.4304, 602.1157) (82.5119, 602.3306) (82.5119, 602.4764) knots 0 0 0 1 2 2 2
  spline S209 degree 2 poles (84.2829, 600.3077) (83.7346, 600.3077) (83.1319, 600.9227) (83.1319, 601.4908) knots 0 0 0 1 2 2 2
  spline S210 degree 2 poles (83.1319, 601.4908) (83.1319, 602.0491) (83.7173, 602.711) (84.1891, 602.711) knots 0 0 0 1 2 2 2
  spline S211 degree 2 poles (84.1891, 602.711) (84.4015, 602.711) (84.73, 602.5875) (84.851, 602.4566) knots 0 0 0 1 2 2 2
  spline S212 degree 2 poles (84.851, 602.4566) (84.9745, 602.3257) (85.1054, 601.9478) (85.1054, 601.6736) knots 0 0 0 1 2 2 2
  line L243 (85.1054, 601.6736) -> (85.1054, 601.4637)
  line L244 (85.1054, 601.4637) -> (83.5221, 601.4637)
  spline S213 degree 2 poles (83.5221, 601.4637) (83.5221, 601.066) (83.9223, 600.6436) (84.278, 600.6436) knots 0 0 0 1 2 2 2
  spline S214 degree 2 poles (84.278, 600.6436) (84.4039, 600.6436) (84.6485, 600.7004) (84.7473, 600.7449) knots 0 0 0 1 2 2 2
  spline S215 degree 2 poles (84.7473, 600.7449) (84.851, 600.7943) (84.9943, 600.8807) (85.0412, 600.9203) knots 0 0 0 1 2 2 2
  line L245 (85.0412, 600.9203) -> (85.0634, 600.9203)
  line L246 (85.0634, 600.9203) -> (85.0634, 600.5004)
  spline S216 degree 2 poles (85.0634, 600.5004) (84.9967, 600.4732) (84.7942, 600.3941) (84.7152, 600.3719) knots 0 0 0 1 2 2 2
  spline S217 degree 2 poles (84.7152, 600.3719) (84.604, 600.3398) (84.4212, 600.3077) (84.2829, 600.3077) knots 0 0 0 1 2 2 2
  spline S218 degree 2 poles (84.73, 601.7576) (84.725, 601.9132) (84.6608, 602.1404) (84.5991, 602.217) knots 0 0 0 1 2 2 2
  spline S219 degree 2 poles (84.5991, 602.217) (84.5324, 602.3035) (84.3224, 602.3949) (84.1668, 602.3949) knots 0 0 0 1 2 2 2
  spline S220 degree 2 poles (84.1668, 602.3949) (84.0137, 602.3949) (83.7988, 602.3035) (83.7099, 602.2145) knots 0 0 0 1 2 2 2
  spline S221 degree 2 poles (83.7099, 602.2145) (83.6234, 602.1232) (83.5345, 601.9033) (83.5221, 601.7576) knots 0 0 0 1 2 2 2
  line L247 (83.5221, 601.7576) -> (84.73, 601.7576)
  line L248 (86.7085, 602.2343) -> (86.6887, 602.2343)
  spline S222 degree 2 poles (86.6887, 602.2343) (86.6442, 602.2467) (86.5479, 602.2516) (86.4812, 602.2516) knots 0 0 0 1 2 2 2
  spline S223 degree 2 poles (86.4812, 602.2516) (86.3256, 602.2516) (86.0193, 602.1157) (85.881, 601.9824) knots 0 0 0 1 2 2 2
  line L249 (85.881, 601.9824) -> (85.881, 600.3596)
  line L250 (85.881, 600.3596) -> (85.4957, 600.3596)
  line L251 (85.4957, 600.3596) -> (85.4957, 602.6468)
  line L252 (85.4957, 602.6468) -> (85.881, 602.6468)
  line L253 (85.881, 602.6468) -> (85.881, 602.3059)
  spline S224 degree 2 poles (85.881, 602.3059) (86.091, 602.4937) (86.4047, 602.6468) (86.5529, 602.6468) knots 0 0 0 1 2 2 2
  spline S225 degree 2 poles (86.5529, 602.6468) (86.6121, 602.6468) (86.6714, 602.6419) (86.7085, 602.6344) knots 0 0 0 1 2 2 2
  line L254 (86.7085, 602.6344) -> (86.7085, 602.2343)
  spline S226 degree 2 poles (87.9163, 600.3077) (87.6792, 600.3077) (87.2865, 600.4534) (87.1457, 600.6016) knots 0 0 0 1 2 2 2
  spline S227 degree 2 poles (87.1457, 600.6016) (87.0049, 600.7474) (86.8493, 601.1969) (86.8493, 601.4982) knots 0 0 0 1 2 2 2
  spline S228 degree 2 poles (86.8493, 601.4982) (86.8493, 601.7996) (87.0098, 602.2392) (87.1457, 602.3874) knots 0 0 0 1 2 2 2
  spline S229 degree 2 poles (87.1457, 602.3874) (87.2815, 602.5381) (87.6841, 602.6987) (87.9163, 602.6987) knots 0 0 0 1 2 2 2
  spline S230 degree 2 poles (87.9163, 602.6987) (88.104, 602.6987) (88.4548, 602.5925) (88.5906, 602.5233) knots 0 0 0 1 2 2 2
  line L255 (88.5906, 602.5233) -> (88.5906, 602.091)
  line L256 (88.5906, 602.091) -> (88.5684, 602.091)
  spline S231 degree 2 poles (88.5684, 602.091) (88.5264, 602.1256) (88.398, 602.2145) (88.3066, 602.2615) knots 0 0 0 1 2 2 2
  spline S232 degree 2 poles (88.3066, 602.2615) (88.2251, 602.301) (88.0077, 602.3627) (87.9089, 602.3627) knots 0 0 0 1 2 2 2
  spline S233 degree 2 poles (87.9089, 602.3627) (87.61, 602.3627) (87.2469, 601.9107) (87.2469, 601.4982) knots 0 0 0 1 2 2 2
  spline S234 degree 2 poles (87.2469, 601.4982) (87.2469, 601.0956) (87.5977, 600.6436) (87.9089, 600.6436) knots 0 0 0 1 2 2 2
  spline S235 degree 2 poles (87.9089, 600.6436) (88.0966, 600.6436) (88.4375, 600.7992) (88.5684, 600.9203) knots 0 0 0 1 2 2 2
  line L257 (88.5684, 600.9203) -> (88.5906, 600.9203)
  line L258 (88.5906, 600.9203) -> (88.5906, 600.488)
  spline S236 degree 2 poles (88.5906, 600.488) (88.5338, 600.4608) (88.3609, 600.3843) (88.2917, 600.367) knots 0 0 0 1 2 2 2
  spline S237 degree 2 poles (88.2917, 600.367) (88.1929, 600.3373) (88.0373, 600.3077) (87.9163, 600.3077) knots 0 0 0 1 2 2 2
  line L259 (90.7198, 600.3596) -> (90.3345, 600.3596)
  line L260 (90.3345, 600.3596) -> (90.3345, 600.6115)
  spline S238 degree 2 poles (90.3345, 600.6115) (90.1566, 600.4559) (89.838, 600.2953) (89.6404, 600.2953) knots 0 0 0 1 2 2 2
  spline S239 degree 2 poles (89.6404, 600.2953) (89.4922, 600.2953) (89.2279, 600.3941) (89.1316, 600.5004) knots 0 0 0 1 2 2 2
  spline S240 degree 2 poles (89.1316, 600.5004) (89.0328, 600.6066) (88.9241, 600.9301) (88.9241, 601.1623) knots 0 0 0 1 2 2 2
  line L261 (88.9241, 601.1623) -> (88.9241, 602.6468)
  line L262 (88.9241, 602.6468) -> (89.3094, 602.6468)
  line L263 (89.3094, 602.6468) -> (89.3094, 601.3426)